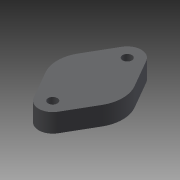
# Autodesk Inventor part: shaftPlug
Saved by Autodesk Inventor 2013 (Build 170138000, 138)
## iProperties
Created: 2015-01-14
Part Number: shaftPlug
Material: Generic
Document SubType Name: Modeling
Designer: dzban
Density: 1 g/cm^3
Author: dzban
Autodesk Inventor part; units mm, degrees
ref_plane "YZ Plane" through (0, 0, 0) normal (1, 0, 0) x (0, 1, 0)
ref_plane "XZ Plane" through (0, 0, 0) normal (0, 1, 0) x (-1, 0, 0)
ref_plane "XY Plane" through (0, 0, 0) normal (0, 0, 1) x (1, 0, 0)
sketch "Sketch1" plane through (0, 0, 0) normal (0, 0, 1) x (1, 0, 0)
  circle A0 centre (0, -12) radius 1.5
  circle A1 centre (0, 12) radius 1.5
  line L0 (3.8971, -14.25) -> (9.0933, -5.25)
  arc A2 (9.0933, -5.25) -> (9.0933, 5.25) centre (0, 0) ccw
  line L1 (9.0933, 5.25) -> (3.8971, 14.25)
  arc A3 (3.8971, 14.25) -> (-3.8971, 14.25) centre (0, 12) ccw
  line L2 (-3.8971, 14.25) -> (-9.0933, 5.25)
  arc A4 (-9.0933, 5.25) -> (-9.0933, -5.25) centre (0, 0) ccw
  line L3 (-9.0933, -5.25) -> (-3.8971, -14.25)
  arc A5 (-3.8971, -14.25) -> (3.8971, -14.25) centre (0, -12) ccw
  constraints: 8 end point, 8 point on circle, 6 centre point
extrude "Extrusion1" add sketch "Sketch1" along normal blind 6
body "Solid1"
